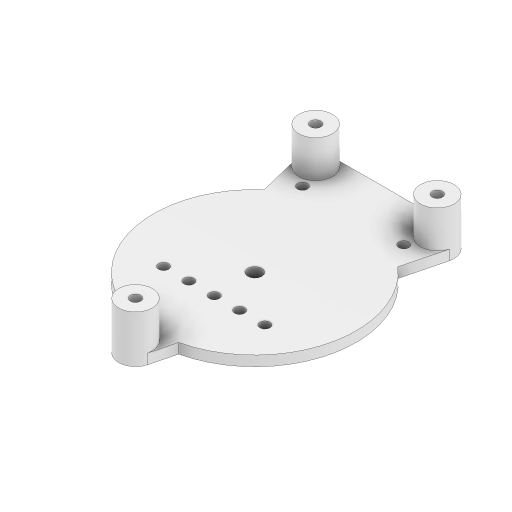
# Autodesk Inventor part: BASE_LIDAR_V3
Saved by Autodesk Inventor 2024.2 (Build 282272000, 272)
## iProperties
Created: 2024-07-17
Part Number: BASE_LIDAR_V3
Material: ABS Plastic
Document SubType Name: Modeling
Designer: jrcer
Density: 1.06 g/cm^3
Appearance: Smooth - White
Author: jrcer
Autodesk Inventor part; units mm, degrees
ref_plane "YZ Plane" through (0, 0, 0) normal (1, 0, 0) x (0, 1, 0)
ref_plane "XZ Plane" through (0, 0, 0) normal (0, 1, 0) x (-1, 0, 0)
ref_plane "XY Plane" through (0, 0, 0) normal (0, 0, 1) x (1, 0, 0)
sketch "Sketch1" plane through (0, 0, 0) normal (0, 1, 0) x (-1, 0, 0)
  circle A0 centre (0, 35.3) radius 1.55
  circle A1 centre (18, -36) radius 1.55
  circle A2 centre (-18, -36) radius 1.55
  circle A3 centre (0, 35.3) radius 5
  circle A4 centre (18, -36) radius 5
  circle A5 centre (-18, -36) radius 5
  point P0 (0, 0)
  dimension "d0" = 35.3
  dimension "d1" = 36
  dimension "d2" = 3.1
  dimension "d3" = 10
  dimension "d4" = 36
  dimension "d5" = 18
  constraints: 6 centre point, 4 equal radius, 3 coincident, 1 horizontal alignment, 1 vertical alignment
  measures "d0" distance of A0.centre point (0, 0)
  measures "d1" vertical distance of A2.centre point (0, 0)
  measures "d2" diameter of A0
  measures "d3" diameter of A3
  measures "d4" distance of A2.centre A1.centre
  measures "d5" horizontal distance of point (0, 0) A2.centre
extrude "Extrusion1" add sketch "Sketch1" along normal blind 11
sketch "Sketch2" plane through (0, 0, 35.3) normal (0, -1, 0) x (1, 0, 0)
  circle A0 centre (0, 0) radius 5 projected
  circle A1 centre (0, 0) radius 1.55 projected
  circle A2 centre (-18, -71.3) radius 1.55 projected
  circle A3 centre (-18, -71.3) radius 5 projected
  circle A4 centre (18, -71.3) radius 1.55 projected
  circle A5 centre (18, -71.3) radius 5 projected
  line L0 (-22.8479, -70.0761) -> (-4.8479, 1.2239)
  line L1 (22.8479, -70.0761) -> (4.8479, 1.2239)
  line L2 (-18, -76.3) -> (18, -76.3)
  circle A6 centre (0, -35.3) radius 2.1
  circle A7 centre (0, -35.3) radius 30
  circle A8 centre (0, -23.3) radius 1.5
  circle A9 centre (-7.5, -23.3) radius 1.5
  circle A10 centre (-15, -23.3) radius 1.5
  circle A11 centre (7.5, -23.3) radius 1.5
  circle A12 centre (15, -23.3) radius 1.5
  circle A13 centre (-15, -64.4) radius 1.5
  circle A14 centre (15, -64.4) radius 1.5
  point P0 (6.6853, -6.0544)
  point P1 (19.7659, -57.8679)
  point P2 (-6.6853, -6.0544)
  point P3 (-19.7659, -57.8679)
  dimension "d8" = 4.2
  dimension "d78" = 60
  dimension "d79" = 12
  dimension "d80" = 7.5
  dimension "d81" = 7.5
  dimension "d82" = 3
  dimension "d83" = 7.5
  dimension "d84" = 7.5
  dimension "d85" = 41.1
  constraints: 9 centre point, 6 end point, 6 equal radius, 6 point on circle, 5 horizontal alignment, 5 tangent, 3 vertical alignment, 2 coincident, 1 horizontal
  measures "d8" diameter of A6
  measures "d78" diameter of A7
  measures "d79" distance of A8.centre point (0, -35.3)
  measures "d80" distance of A8.centre A9.centre
  measures "d81" distance of A10.centre A9.centre
  measures "d82" diameter of A8
  measures "d83" distance of A11.centre A8.centre
  measures "d84" distance of A11.centre A12.centre
  measures "d85" distance of A10.centre A13.centre
extrude "Extrusion2" add sketch "Sketch2" along normal blind 3
equation "\"d5\" = 0.5 * d4"
body "Solid1"
